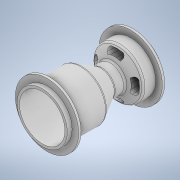
# Autodesk Inventor part: Trục dẫn bánh răng
Saved by Autodesk Inventor 2022 (Build 260153000, 153)
## iProperties
Created: 2022-04-22
Part Number: Trục dẫn bánh răng
Material: Generic
Document SubType Name: Modeling
Designer: duyne
Density: 1 g/cm^3
Appearance: Default
Author: duyne
Autodesk Inventor part; units mm, degrees
ref_plane "YZ Plane" through (0, 0, 0) normal (1, 0, 0) x (0, 1, 0)
ref_plane "XZ Plane" through (0, 0, 0) normal (0, 1, 0) x (-1, 0, 0)
ref_plane "XY Plane" through (0, 0, 0) normal (0, 0, 1) x (1, 0, 0)
sketch "Sketch1" plane through (0, 0, 0) normal (1, 0, 0) x (0, 1, 0)
  line L0 (10.5, 18.8712) -> (10.5, 16.8712)
  line L1 (10.5, 16.8712) -> (13.25, 16.8712)
  line L2 (13.25, 16.8712) -> (13.25, 15.8712)
  line L3 (13.25, 15.8712) -> (10.5, 15.8712)
  line L4 (10.5, 15.8712) -> (10.5, 2.8712)
  line L5 (10.364, 2.3677) -> (5.716, -5.6092)
  line L6 (5.58, -6.1126) -> (5.58, -9.6126)
  line L7 (6.0765, -10.4766) -> (10.0035, -12.7648)
  line L8 (10.5, -13.6288) -> (10.5, -18.1288)
  line L9 (10.5, -18.1288) -> (13.25, -18.1288)
  line L10 (13.25, -18.1288) -> (13.25, -19.1288)
  line L11 (13.25, -19.1288) -> (10.5, -19.1288)
  line L12 (10.5, -19.1288) -> (10.5, -21.1288)
  line L13 (10.5, -21.1288) -> (0, -21.1288)
  line L14 (10.5, 18.8712) -> (0, 18.8712)
  line L15 (0, 27.6425) -> (0, -28.3575) projected
  arc A0 (10.364, 2.3677) -> (10.5, 2.8712) centre (9.5, 2.8712) ccw
  arc A1 (5.716, -5.6092) -> (5.58, -6.1126) centre (6.58, -6.1126) ccw
  arc A2 (5.58, -9.6126) -> (6.0765, -10.4766) centre (6.58, -9.6126) ccw
  arc A3 (10.5, -13.6288) -> (10.0035, -12.7648) centre (9.5, -13.6288) ccw
  point P0 (0, 0)
  point P1 (10.5, 2.6011)
  point P2 (5.58, -5.8425)
  dimension "d0" = 10.5
  dimension "d1" = 2
  dimension "d2" = 13.25
  dimension "d4" = 10.5
  dimension "d5" = 5.58
  dimension "d6" = 0
  dimension "d7" = 10.5
  dimension "d8" = 13.25
  dimension "d9" = 1
  dimension "d10" = 1
  dimension "d11" = 1
  dimension "d13" = 13
  dimension "d14" = 1
  dimension "d15" = 3.5
  dimension "d16" = 4.5
  dimension "d17" = 1
  dimension "d18" = 2
  dimension "d40" = 40
  constraints: 30 end point, 8 perpendicular, 8 point on circle, 8 point on line, 8 tangent, 4 centre point, 1 collinear, 1 equal radius, 1 horizontal, 1 parallel, 1 vertical
  measures "d0" distance of L0.start L14.end
  measures "d1" distance of L0.start L0.end
  measures "d2" distance from line of L15 L1.end
  measures "d4" distance between parallel lines of L15 L4
  measures "d5" distance from line of L15 point (5.58, -5.843)
  measures "d6" distance from line of L15 L13.end
  measures "d7" distance between parallel lines of L15 L8
  measures "d8" distance between parallel lines of L15 L10
  measures "d9" radius of A0
  measures "d10" radius of A1
  measures "d11" radius of A2
  measures "d13" distance of L3.end L4.end
  measures "d14" distance of L1.end L2.end
  measures "d15" distance of L6.start L6.end
  measures "d16" distance of L8.start L8.end
  measures "d17" distance of L9.end L10.end
  measures "d18" distance of L11.end L12.end
  measures "d40" distance between parallel lines of L13 L14
revolve "Revolution1" add sketch "Sketch1" angle 360 about axis through (0, 0, 0) along (0, 0, -1)
sketch "Sketch6" plane through (0, 0, -21.1288) normal (0, 0, -1) x (-1, 0, 0)
  circle A0 centre (0, 0) radius 4
  dimension "d19" = 8
  constraints: 1 centre point, 1 coincident
  measures "d19" diameter of A0
extrude "Extrusion1" cut sketch "Sketch6" against normal through all
sketch "Sketch7" plane through (0, 0, 18.8712) normal (0, 0, 1) x (1, 0, 0)
  circle A0 centre (0, 0) radius 9.5
  dimension "d22" = 19
  constraints: 1 centre point, 1 coincident
  measures "d22" diameter of A0
extrude "Extrusion2" cut sketch "Sketch7" against normal blind 15
sketch "Sketch8" plane through (0, 0, -21.1288) normal (0, 0, -1) x (-1, 0, 0)
  circle A0 centre (0, 0) radius 9.5
  dimension "d25" = 19
  constraints: 1 centre point, 1 coincident
  measures "d25" diameter of A0
extrude "Extrusion3" cut sketch "Sketch8" against normal blind 5
sketch "Sketch9" plane through (0, 0, -16.1288) normal (0, 0, -1) x (-1, 0, 0)
  circle A0 centre (0, 0) radius 5.5
  dimension "d28" = 11
  constraints: 1 centre point, 1 coincident
  measures "d28" diameter of A0
extrude "Extrusion4" add sketch "Sketch9" along normal blind 1.8
sketch "Sketch10" plane through (0, 0, -17.9288) normal (0, 0, -1) x (-1, 0, 0)
  circle A0 centre (0, 0) radius 4
  dimension "d31" = 8
  constraints: 1 centre point, 1 coincident
  measures "d31" diameter of A0
extrude "Extrusion5" cut sketch "Sketch10" against normal blind 19.491
sketch "Sketch11" plane through (0, 0, -16.1288) normal (0, 0, -1) x (-1, 0, 0)
  circle A0 centre (0, 0) radius 5.5 projected
  arc A1 (0, 5.5) -> (2.3061, 6.1198) centre (0.5248, 8.1473) ccw
  line L0 (2.3061, 6.1198) -> (3.0697, 7.2802)
  arc A2 (3.0697, 7.2802) -> (2.3061, 9.2056) centre (2.0133, 7.9754) ccw
  line L1 (2.3061, 9.2056) -> (0, 9.4677)
  circle A3 centre (0, 0) radius 10.0035 projected
  arc A4 (-2.3061, 6.1198) -> (0, 5.5) centre (-0.5248, 8.1473) ccw
  line L2 (-2.3061, 6.1198) -> (-3.0697, 7.2802)
  arc A5 (-2.3061, 9.2056) -> (-3.0697, 7.2802) centre (-2.0133, 7.9754) ccw
  line L3 (-2.3061, 9.2056) -> (0, 9.4677)
  point P0 (-0.7056, 5.4545)
  point P1 (0.7056, 5.4545)
  dimension "d34" = 1.2645
  constraints: 8 end point, 8 point on circle, 4 centre point, 1 tangent, 2 other
  measures "d34" radius of A2
extrude "Extrusion6" cut sketch "Sketch11" against normal blind 4.991 contours A0 A4 L2 A5 L3 L1 A2 L0 A1
pattern_circular "Circular Pattern1" count 4 over 360 about axis through (0, 0, -11.6207) along (0, 0, -1) of "Extrusion6"
fillet "Fillet1" radius 1 1 edges at (0, -10.5, 15.8712)
body "Solid1"
